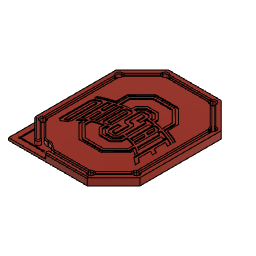
blockO_model (Autodesk Fusion 360 design; units mm, degrees)
Autodesk Fusion 360 part; units mm, degrees
(part 1 of 2)
sketch "Sketch1" plane through (0, 0, 0) normal (0, 0, 1) x (1, 0, 0)
  line L0 (0, 0) -> (25, 0)
  line L1 (0, 0) -> (-24, 24)
  line L2 (-24, 24) -> (-24, 104)
  line L3 (-24, 104) -> (0, 128)
  line L4 (0, 128) -> (25, 128)
  line L5 (25, 128) -> (25, 0) construction
  line L6 (50, 128) -> (25, 128)
  line L7 (74, 104) -> (50, 128)
  line L8 (74, 24) -> (74, 104)
  line L9 (50, 0) -> (74, 24)
  line L10 (50, 0) -> (25, 0)
  line L11 (0.4142, 127) -> (25, 127)
  line L12 (49.5858, 127) -> (25, 127)
  line L13 (73, 103.5858) -> (49.5858, 127)
  line L14 (73, 24.4142) -> (73, 103.5858)
  line L15 (49.5858, 1) -> (73, 24.4142)
  line L16 (49.5858, 1) -> (25, 1)
  line L17 (0.4142, 1) -> (25, 1)
  line L18 (0.4142, 1) -> (-23, 24.4142)
  line L19 (-23, 24.4142) -> (-23, 103.5858)
  line L20 (-23, 103.5858) -> (0.4142, 127)
  line L21 (50.4142, 129) -> (25, 129)
  line L22 (-0.4142, 129) -> (25, 129)
  line L23 (-25, 104.4142) -> (-0.4142, 129)
  line L24 (-25, 23.5858) -> (-25, 104.4142)
  line L25 (-0.4142, -1) -> (-25, 23.5858)
  line L26 (-0.4142, -1) -> (25, -1)
  line L27 (50.4142, -1) -> (25, -1)
  line L28 (50.4142, -1) -> (75, 23.5858)
  line L29 (75, 23.5858) -> (75, 104.4142)
  line L30 (75, 104.4142) -> (50.4142, 129)
  line L31 (-2.4853, 134) -> (25, 134)
  line L32 (52.4853, 134) -> (25, 134)
  line L33 (80, 106.4853) -> (52.4853, 134)
  line L34 (80, 21.5147) -> (80, 106.4853)
  line L35 (52.4853, -6) -> (80, 21.5147)
  line L36 (52.4853, -6) -> (25, -6)
  line L37 (-2.4853, -6) -> (25, -6)
  line L38 (-2.4853, -6) -> (-30, 21.5147)
  line L39 (-30, 21.5147) -> (-30, 106.4853)
  line L40 (-30, 106.4853) -> (-2.4853, 134)
  line L41 (-30, 21.5147) -> (-30, -6)
  line L42 (-30, -6) -> (-2.4853, -6)
  circle A0 centre (-24, 24) radius 2.5
  circle A1 centre (-24, 104) radius 2.5
  circle A2 centre (0, 128) radius 2.5
  circle A3 centre (50, 128) radius 2.5
  circle A4 centre (74, 104) radius 2.5
  circle A5 centre (74, 24) radius 2.5
  circle A6 centre (50, 0) radius 2.5
  circle A7 centre (0, 0) radius 6.4944
  line L43 (-4.5922, 4.5922) -> (-8.8348, 0.3496)
  line L44 (6.4944, 0) -> (6.4944, -6)
  line L45 (46.8934, 7.5) -> (25, 7.5)
  line L46 (3.1066, 7.5) -> (25, 7.5)
  line L47 (3.1066, 7.5) -> (-16.5, 27.1066)
  line L48 (-16.5, 27.1066) -> (-16.5, 100.8934)
  line L49 (-16.5, 100.8934) -> (3.1066, 120.5)
  line L50 (3.1066, 120.5) -> (25, 120.5)
  line L51 (46.8934, 120.5) -> (25, 120.5)
  line L52 (66.5, 100.8934) -> (46.8934, 120.5)
  line L53 (66.5, 27.1066) -> (66.5, 100.8934)
  line L54 (46.8934, 7.5) -> (66.5, 27.1066)
  line L55 (45.8579, 10) -> (25, 10)
  line L56 (4.1421, 10) -> (25, 10)
  line L57 (4.1421, 10) -> (-14, 28.1421)
  line L58 (-14, 28.1421) -> (-14, 99.8579)
  line L59 (-14, 99.8579) -> (4.1421, 118)
  line L60 (4.1421, 118) -> (25, 118)
  line L61 (45.8579, 118) -> (25, 118)
  line L62 (64, 99.8579) -> (45.8579, 118)
  line L63 (64, 28.1421) -> (64, 99.8579)
  line L64 (45.8579, 10) -> (64, 28.1421)
  line L65 (38.7955, 27.05) -> (25, 27.05)
  line L66 (11.2045, 27.05) -> (25, 27.05)
  line L67 (11.2045, 27.05) -> (3.05, 35.2045)
  line L68 (3.05, 35.2045) -> (3.05, 92.7955)
  line L69 (3.05, 92.7955) -> (11.2045, 100.95)
  line L70 (11.2045, 100.95) -> (25, 100.95)
  line L71 (38.7955, 100.95) -> (25, 100.95)
  line L72 (46.95, 92.7955) -> (38.7955, 100.95)
  line L73 (46.95, 35.2045) -> (46.95, 92.7955)
  line L74 (38.7955, 27.05) -> (46.95, 35.2045)
  line L75 (12.4885, 30.15) -> (25, 30.15)
  line L76 (37.5115, 30.15) -> (25, 30.15)
  line L77 (37.5115, 30.15) -> (43.85, 36.4885)
  line L78 (43.85, 36.4885) -> (43.85, 91.5115)
  line L79 (43.85, 91.5115) -> (37.5115, 97.85)
  line L80 (37.5115, 97.85) -> (25, 97.85)
  line L81 (12.4885, 97.85) -> (25, 97.85)
  line L82 (6.15, 91.5115) -> (12.4885, 97.85)
  line L83 (6.15, 36.4885) -> (6.15, 91.5115)
  line L84 (12.4885, 30.15) -> (6.15, 36.4885)
  line L85 (36.4759, 32.65) -> (25, 32.65)
  line L86 (13.5241, 32.65) -> (25, 32.65)
  line L87 (13.5241, 32.65) -> (8.65, 37.5241)
  line L88 (8.65, 37.5241) -> (8.65, 90.4759)
  line L89 (8.65, 90.4759) -> (13.5241, 95.35)
  line L90 (13.5241, 95.35) -> (25, 95.35)
  line L91 (36.4759, 95.35) -> (25, 95.35)
  line L92 (41.35, 90.4759) -> (36.4759, 95.35)
  line L93 (41.35, 37.5241) -> (41.35, 90.4759)
  line L94 (36.4759, 32.65) -> (41.35, 37.5241)
  line L95 (-23, 24.4142) -> (-25, 24.4142)
  line L96 (-25, 24.4142) -> (-23, 24.4142)
  line L97 (-23, 24.4142) -> (-23, 1)
  line L98 (-25, -1) -> (-25, 24.4142)
  line L99 (-0.4142, -1) -> (-25, -1)
  line L100 (-25, -1) -> (-25, 1)
  line L101 (-23, 1) -> (-0.4142, 1)
  line L102 (-0.4142, 1) -> (-0.4142, -1)
  line L103 (-24.5, -0.5) -> (-24.5, 23.9142)
  line L104 (-24.5, 23.9142) -> (-23.5, 23.9142)
  line L105 (-23.5, 23.9142) -> (-23.5, 0.5)
  line L106 (-23.5, 0.5) -> (-0.9142, 0.5)
  line L107 (-0.9142, 0.5) -> (-0.9142, -0.5)
  line L108 (-0.9142, -0.5) -> (-24.5, -0.5)
  line L109 (0, 0) -> (-51.0387, 0) construction
  line L110 (-24, 24) -> (-24, -3.1074) construction
  circle A8 centre (-24, 0) radius 1
  circle A9 centre (0, 0) radius 1.0824
  spline S0 degree 3 poles (-34.7934, -51.0937) (-33.9487, -51.2384) (-33.2949, -51.3375) (-32.4316, -51.4451) knots 0 0 0 0 1 1 1 1
  constraint coincident L0.start L1.start
  constraint horizontal L0
  constraint vertical L2
  constraint perpendicular L2 L4
  constraint symmetric L0.start L5 L9.start
  constraint symmetric L0.end L5 L10.end
  constraint symmetric L1.end L5 L8.start
  constraint symmetric L2.end L5 L7.start
  constraint symmetric L3.end L5 L6.start
  constraint symmetric L4.end L5 L6.end
  constraint perpendicular L37 L41
  constraint perpendicular L39 L42
  constraint coincident L1.end L2.start
  constraint coincident L2.end L3.start
  constraint coincident L3.end L4.start
  constraint coincident L6.start L7.end
  constraint coincident L7.start L8.end
  constraint coincident L8.start L9.end
  constraint coincident L9.start L10.start
  constraint equal A0 A1
  constraint equal A2 A3
  constraint equal A3 A4
  constraint equal A4 A5
  constraint equal A5 A6
  constraint coincident L37.start A7
  constraint coincident A7 L43.start
  constraint coincident L1 L43.start
  constraint coincident L38 L43.end
  constraint tangent A7 L43
  constraint coincident A7 L44.start
  constraint coincident L0 L44.start
  constraint coincident L37 L44.end
  constraint tangent A7 L44
  constraint equal A1 A2
  constraint coincident L24 L95.end
  constraint perpendicular L24 L95
  constraint horizontal L96
  constraint vertical L97
  constraint vertical L98
  constraint horizontal L99
  constraint vertical L100
  constraint horizontal L101
  constraint vertical L102
  constraint coincident L98 L100.end
  constraint collinear L17 L101
  constraint collinear L19 L97
  constraint perpendicular L98 L109
  constraint parallel L105 L110
  constraint coincident L109 A8.centre
  constraint coincident L110 A8.centre
  constraint tangent L99 A8
  constraint concentric A7 A9
  constraint coincident L101.end A9
extrude "Extrude1" add sketch "Sketch1" against normal blind 5 contours L17 L18 A7 | L26 A9 | L26 L37 L38 A7 L99 A9 | L25 L108 A9 | A7 L99 L108 A9 | L11 L12 L13 L14 L15 L16 L17 L18 L19 L20 A0 A1 A2 A3 A4 A5 A6 A7 | L26 L37 A7 L44 | L21 L22 L23 L24 L26 L27 L28 L29 L30 L31 L32 L33 L34 L35 L36 L37 L38 L39 L40 A0 A1 A2 A3 A4 A5 A6 L44 L98 | L25 L108 A9 | L38 A7 L99 L108 | L38 A7 L99 | L25 A7 L106 L108 A9 | L18 L19 A0 | L25 A7 L101 | L25 A7 L101 L106 | L38 A7 L43 L106 L108 | L15 L16 A6 | L27 L28 A6 | L25 A7 L43 L101 | L25 L38 L43 L97 L101 | A7 L43 L101 L106 | L25 L38 A0 L97 L105 | L38 L43 L101 L106 | L38 L43 L106 | L14 L15 A5 | L19 L20 A1 | L24 A0 L98 | L25 A0 L105 | L28 L29 A5 | L38 A0 L98 L103 | L25 A0 L98 L103 | L25 A0 L103 L105 | L38 A0 L103 L105 | L13 L14 A4 | L23 L24 A1 | L11 L20 A2 | L29 L30 A4 | L12 L13 A3 | L22 L23 A2 | L21 L30 A3 | L45 L46 L47 L48 L49 L50 L51 L52 L53 L54 | L55 L56 L57 L58 L59 L60 L61 L62 L63 L64 | L65 L66 L67 L68 L69 L70 L71 L72 L73 L74 | L75 L76 L77 L78 L79 L80 L81 L82 L83 L84 | L85 L86 L87 L88 L89 L90 L91 L92 L93 L94 makes body 1 at (9, 77.1953, -5) makes body 2 at (78.3333, 50.5286, -5)
sketch "Sketch3" plane through (0, 0, -5) normal (0, 0, -1) x (1, 0, 0)
  line L0 (49.5858, -1) -> (0.4142, -1)
  line L1 (0.4142, -1) -> (-23, -24.4142)
  line L2 (-23, -24.4142) -> (-23, -103.5858)
  line L3 (-23, -103.5858) -> (0.4142, -127)
  line L4 (0.4142, -127) -> (49.5858, -127)
  line L5 (49.5858, -127) -> (73, -103.5858)
  line L6 (73, -103.5858) -> (73, -24.4142)
  line L7 (73, -24.4142) -> (49.5858, -1)
  line L8 (52.4853, -134) -> (80, -106.4853)
  line L9 (-2.4853, -134) -> (52.4853, -134)
  line L10 (-30, -106.4853) -> (-2.4853, -134)
  line L11 (-30, -21.5147) -> (-30, -106.4853)
  line L12 (-2.4853, 6) -> (-30, -21.5147)
  line L13 (52.4853, 6) -> (-2.4853, 6)
  line L14 (80, -21.5147) -> (52.4853, 6)
  line L15 (80, -106.4853) -> (80, -21.5147)
  line L16 (-30, -21.5147) -> (-30, 6)
  line L17 (-30, 6) -> (-2.4853, 6)
  constraint coincident L11.start L12.end
  constraint perpendicular L13 L16
  constraint coincident L12.start L13.end
  constraint perpendicular L16 L17
extrude "Extrude2" add sketch "Sketch3" along normal blind 2.5 contours L0 L1 L2 L3 L4 L5 L6 L7 | L8 L9 L10 L11 L12 L13 L14 L15 bodies 1 2
extrude "Extrude3" add sketch "Sketch3" along normal blind 2.5 contours L12 L16 L17 bodies 1
sketch "Sketch4" plane through (0, 0, 0) normal (0, 0, 1) x (1, 0, 0)
extrude "Extrude4" cut sketch "Sketch1" against normal up to surface (5 mm away) contours L9 L10 L15 L16 A6 | L9 L10 L27 L28 A6 | L1 L18 A0 L97 | L18 L19 A0 | L15 L16 A6 | L27 L28 A6 | L2 L19 A0 L95 L96 | L1 L2 L95 L96 L97 L104 L105 | L1 A0 L97 | L2 L24 A0 L95 L96 | L1 L2 L24 L25 L95 L96 L98 L103 L104 | L1 L25 A0 L97 L105 | L8 L9 L14 L15 A5 | L8 L9 L28 L29 A5 | L14 L15 A5 | L2 L3 L19 L20 A1 | L19 L20 A1 | L24 A0 L98 | L1 L25 L103 L104 L105 | L1 L104 L105 | L25 A0 L105 | L28 L29 A5 | L2 L3 L23 L24 A1 | L25 A0 L98 L103 | L25 A0 L103 L105 | L13 L14 A4 | L7 L8 L13 L14 A4 | L23 L24 A1 | L7 L8 L29 L30 A4 | L3 L4 L11 L20 A2 | L11 L20 A2 | L29 L30 A4 | L12 L13 A3 | L6 L7 L12 L13 A3 | L3 L4 L22 L23 A2 | L22 L23 A2 | L6 L7 L21 L30 A3 | L21 L30 A3 bodies 1
extrude "Extrude5" cut sketch "Sketch1" against normal up to surface (5 mm away) contours L17 L18 A7 | L26 A9 | L26 L37 L38 A7 L99 A9 | L25 L108 A9 | A7 L99 L108 A9 | L26 L37 A7 L44 | L25 L108 A9 | L38 A7 L99 L108 | L38 A7 L99 | L25 A7 L106 L108 A9 | L25 A7 L101 | L25 A7 L101 L106 | L38 A7 L43 L106 L108 | L25 A7 L43 L101 | A7 L43 L101 L106 bodies 1
fillet "Fillet1" radius 7 2 edges at (-3.8303, 5.2445, -2.5) (6.4169, 1, -2.5) on bodies 1
fillet "Fillet2" radius 2.5 4 edges at (-5.2993, 3.8851, -2.5) (-8.8348, 0.3496, -2.5) (6.4944, -6, -2.5) (6.4944, -1, -2.5) on bodies 1
fillet "Fillet3" radius 2.5 28 edges at (-23, 26.2913, -2.5) (-21.6727, 23.0869, -2.5) (-25, 26.2913, -2.5) (-23.0869, 21.6727, -2.5) (-23.0869, 106.3273, -2.5) (-21.6727, 104.9131, -2.5) (-25, 101.7087, -2.5) (-23, 101.7087, -2.5) (2.2913, 129, -2.5) (-2.3273, 127.0869, -2.5) (-0.9131, 125.6727, -2.5) (2.2913, 127, -2.5) (52.3273, 127.0869, -2.5) (47.7087, 129, -2.5) (47.7087, 127, -2.5) (50.9131, 125.6727, -2.5) (73.0869, 106.3273, -2.5) (71.6727, 104.9131, -2.5) (73, 101.7087, -2.5) (75, 101.7087, -2.5) (73, 26.2913, -2.5) (71.6727, 23.0869, -2.5) (73.0869, 21.6727, -2.5) (75, 26.2913, -2.5) (50.9131, 2.3273, -2.5) (47.7087, 1, -2.5) (47.7087, -1, -2.5) (52.3273, 0.9131, -2.5) on bodies 1
fillet "Fillet4" radius 1 65 edges at (71.3147, 23.0049, 0) (71.6903, 24.9567, 0) (72.8049, 26.6025, 0) (73, 64, 0) (72.8049, 101.3975, 0) (71.6903, 103.0433, 0) (71.3147, 104.9951, 0) (61.2929, 115.2929, 0) (50.9951, 125.3147, 0) (49.0433, 125.6903, 0) (47.3975, 126.8049, 0) (25, 127, 0) (2.6025, 126.8049, 0) (0.9567, 125.6903, 0) (-0.9951, 125.3147, 0) (-11.2929, 115.2929, 0) (-21.3147, 104.9951, 0) (-21.6903, 103.0433, 0) (-22.8049, 101.3975, 0) (-23, 64, 0) (-22.8049, 26.6025, 0) (-21.6903, 24.9567, 0) (-21.3147, 23.0049, 0) (-13.8726, 15.2868, 0) (-4.2114, 6.6906, 0) (2.4853, 6, 0) (7.7089, 1.753, 0) (28.6483, 1, 0) (47.3975, 1.1951, 0) (49.0433, 2.3097, 0) (50.9951, 2.6853, 0) (61.2929, 12.7071, 0) (-20.3013, 11.816, 0) (-7.0671, 2.1173, 0) (-14.6247, 13.2104, 0) (-23.0049, 21.3147, 0) (-26.3097, 23.0433, 0) (-25.1951, 26.6025, 0) (-25, 64, 0) (-25.1951, 101.3975, 0) (-26.3097, 104.9567, 0) (-23.0049, 106.6853, 0) (-12.7071, 116.7071, 0) (-2.6853, 127.0049, 0) (-0.9567, 130.3097, 0) (2.6025, 129.1951, 0) (25, 129, 0) (47.3975, 129.1951, 0) (50.9567, 130.3097, 0) (52.6853, 127.0049, 0) (62.7071, 116.7071, 0) (73.0049, 106.6853, 0) (76.3097, 104.9567, 0) (75.1951, 101.3975, 0) (75, 64, 0) (75.1951, 26.6025, 0) (76.3097, 23.0433, 0) (73.0049, 21.3147, 0) (62.7071, 11.2929, 0) (52.6853, 0.9951, 0) (50.9567, -2.3097, 0) (47.3975, -1.1951, 0) (27.7118, -1, 0) (6.4944, -3.5, 0) (30.7398, -6, 0) on bodies 1
sketch "Sketch5" plane through (0, 0, 0) normal (0, 0, 1) x (-1, 0, 0)
  arc A0 (-70.0609, -22.8893) -> (-70.5002, -23.965) centre (-69.0003, -23.95) ccw
  arc A1 (-71.55, -26.4995) -> (-70.5002, -23.965) centre (-74, -24) ccw
  arc A2 (-71.55, -26.4995) -> (-72, -27.5707) centre (-70.5, -27.5707) ccw
  line L0 (-72, -27.5707) -> (-72, -100.4293)
  arc A3 (-72, -100.4293) -> (-71.55, -101.5005) centre (-70.5, -100.4293) ccw
  arc A4 (-70.5002, -104.035) -> (-71.55, -101.5005) centre (-74, -104) ccw
  arc A5 (-70.5002, -104.035) -> (-70.0609, -105.1107) centre (-69.0003, -104.05) ccw
  line L1 (-70.0609, -105.1107) -> (-51.1107, -124.0609)
  arc A6 (-51.1107, -124.0609) -> (-50.035, -124.5002) centre (-50.05, -123.0003) ccw
  arc A7 (-47.5005, -125.55) -> (-50.035, -124.5002) centre (-50, -128) ccw
  arc A8 (-47.5005, -125.55) -> (-46.4293, -126) centre (-46.4293, -124.5) ccw
  line L2 (-46.4293, -126) -> (-3.5707, -126)
  arc A9 (-3.5707, -126) -> (-2.4995, -125.55) centre (-3.5707, -124.5) ccw
  arc A10 (0.035, -124.5002) -> (-2.4995, -125.55) centre (0, -128) ccw
  arc A11 (0.035, -124.5002) -> (1.1107, -124.0609) centre (0.05, -123.0003) ccw
  line L3 (1.1107, -124.0609) -> (20.0609, -105.1107)
  arc A12 (20.0609, -105.1107) -> (20.5002, -104.035) centre (19.0003, -104.05) ccw
  arc A13 (21.55, -101.5005) -> (20.5002, -104.035) centre (24, -104) ccw
  arc A14 (21.55, -101.5005) -> (22, -100.4293) centre (20.5, -100.4293) ccw
  line L4 (22, -100.4293) -> (22, -27.5707)
  arc A15 (22, -27.5707) -> (21.55, -26.4995) centre (20.5, -27.5707) ccw
  arc A16 (20.5002, -23.965) -> (21.55, -26.4995) centre (24, -24) ccw
  arc A17 (20.5002, -23.965) -> (20.0609, -22.8893) centre (19.0003, -23.95) ccw
  line L5 (20.0609, -22.8893) -> (6.2701, -9.0985)
  arc A18 (6.2701, -9.0985) -> (1.126, -7.4093) centre (2.0275, -13.3412) ccw
  arc A19 (-6.0354, -4.443) -> (1.126, -7.4093) centre (0, 0) ccw
  arc A20 (-6.0354, -4.443) -> (-10.8673, -2) centre (-10.8673, -8) ccw
  line L6 (-10.8673, -2) -> (-46.4293, -2)
  arc A21 (-46.4293, -2) -> (-47.5005, -2.45) centre (-46.4293, -3.5) ccw
  arc A22 (-50.035, -3.4998) -> (-47.5005, -2.45) centre (-50, 0) ccw
  arc A23 (-50.035, -3.4998) -> (-51.1107, -3.9391) centre (-50.05, -4.9997) ccw
  line L7 (-51.1107, -3.9391) -> (-70.0609, -22.8893)
  line L8 (-108.9308, -166.2766) -> (-108.9012, -188.3914)
  line L9 (-108.9012, -188.3914) -> (-76.1248, -221.0889)
  line L10 (-76.1248, -221.0889) -> (-24.7372, -221.0889)
  line L11 (-24.7372, -221.0889) -> (8.4567, -188.4977)
  line L12 (8.4567, -188.4977) -> (8.4113, -166.3147)
  spline S0 degree 2 poles (8.4113, -166.3147) (24.5675, -160.7554) (37.454, -154.104) knots 0 0 0 1 1 1
  line L13 (37.454, -154.104) -> (37.5982, -69.2711)
  line L14 (37.5982, -69.2711) -> (27.8603, -62.9385)
  line L15 (27.8603, -62.9385) -> (14.9977, -70.6994)
  line L16 (14.9977, -70.6994) -> (9.072, -82.1954)
  line L17 (9.072, -82.1954) -> (-24.7992, -49.3035)
  line L18 (-24.7992, -49.3035) -> (-75.9426, -49.4418)
  line L19 (-75.9426, -49.4418) -> (-102.2338, -75.588)
  spline S1 degree 3 poles (-102.2338, -75.588) (-103.4051, -73.9683) (-105.3092, -72.9156) (-107.482, -72.9156) knots 0 0 0 0 1 1 1 1
  spline S2 degree 3 poles (-107.482, -72.9156) (-109.9076, -72.9156) (-112.0093, -74.237) (-113.1173, -76.1964) knots 0 0 0 0 1 1 1 1
  spline S3 degree 2 poles (-113.1173, -76.1964) (-120.0682, -70.9562) (-136.9942, -57.3225) knots 0 0 0 1 1 1
  line L20 (-136.9942, -57.3225) -> (-137.014, -154.3287)
  spline S4 degree 2 poles (-137.014, -154.3287) (-120.3333, -162.6226) (-108.9324, -166.2753) knots 0 0 0 1 1 1
  line L21 (-44.6848, -172.5597) -> (-40.0611, -168.0135)
  line L22 (-40.0611, -168.0135) -> (-40.0611, -137.1508)
  line L23 (-40.0611, -137.1508) -> (-45.0799, -132.3817)
  line L24 (-45.0799, -132.3817) -> (-53.5181, -132.3817)
  line L25 (-53.5181, -132.3817) -> (-53.5797, -104.2465)
  line L26 (-53.5797, -104.2465) -> (-46.7959, -104.2465)
  line L27 (-46.7959, -104.2465) -> (-46.7959, -123.1725)
  line L28 (-46.7959, -123.1725) -> (-40.0611, -123.1725)
  line L29 (-40.0611, -123.1725) -> (-40.0611, -102.4906)
  line L30 (-40.0611, -102.4906) -> (-44.6973, -97.9317)
  line L31 (-44.6973, -97.9317) -> (-55.9687, -97.8606)
  line L32 (-55.9687, -97.8606) -> (-60.545, -102.4905)
  line L33 (-60.545, -102.4905) -> (-60.4155, -135.4901)
  line L34 (-60.4155, -135.4901) -> (-55.4773, -140.2244)
  line L35 (-55.4773, -140.2244) -> (-46.9631, -140.218)
  line L36 (-46.9631, -140.218) -> (-46.941, -165.5468)
  line L37 (-46.941, -165.5468) -> (-53.7548, -165.5168)
  line L38 (-53.7548, -165.5168) -> (-53.7705, -149.2768)
  line L39 (-53.7705, -149.2768) -> (-60.4532, -149.2879)
  line L40 (-60.4532, -149.2879) -> (-60.4737, -168.035)
  line L41 (-60.4737, -168.035) -> (-55.9339, -172.5591)
  line L42 (-55.9339, -172.5591) -> (-44.6843, -172.5591)
  line L43 (-44.6843, -172.5591) -> (-44.6848, -172.5597)
  line L44 (-61.9499, -162.6549) -> (-61.9625, -156.2109)
  spline S5 degree 2 poles (-61.9625, -156.2109) (-63.7987, -156.0339) (-66.6067, -155.7179) knots 0 0 0 1 1 1
  line L45 (-66.6067, -155.7179) -> (-66.6004, -112.1784)
  spline S6 degree 3 poles (-66.6004, -112.1784) (-68.8917, -111.8466) (-71.2841, -111.5542) (-73.3668, -111.1845) knots 0 0 0 0 1 1 1 1
  line L46 (-73.3668, -111.1845) -> (-73.1556, -154.9169)
  spline S7 degree 2 poles (-73.1556, -154.9169) (-75.7123, -154.5566) (-78.0431, -154.1568) knots 0 0 0 1 1 1
  line L47 (-78.0431, -154.1568) -> (-78.0431, -160.6609)
  spline S8 degree 3 poles (-78.0431, -160.6609) (-72.4903, -161.6422) (-67.53, -162.1637) (-61.9453, -162.6567) knots 0 0 0 0 1 1 1 1
  line L48 (-61.9453, -162.6567) -> (-61.9499, -162.6549)
  spline S9 degree 3 poles (-30.7408, -161.8474) (-27.8253, -161.4571) (-24.8909, -161.1063) (-21.9484, -160.5564) knots 0 0 0 0 1 1 1 1
  line L49 (-21.9484, -160.5564) -> (-18.2902, -155.751)
  line L50 (-18.2902, -155.751) -> (-18.3455, -112.9846)
  line L51 (-18.3455, -112.9846) -> (-21.6576, -110.0059)
  spline S10 degree 3 poles (-21.6576, -110.0059) (-25.4027, -110.9082) (-28.2075, -111.3649) (-31.8243, -111.9196) knots 0 0 0 0 1 1 1 1
  line L52 (-31.8243, -111.9196) -> (-34.8567, -115.9064)
  line L53 (-34.8567, -115.9064) -> (-34.9926, -157.6681)
  line L54 (-34.9926, -157.6681) -> (-30.7404, -161.8477)
  line L55 (-30.7404, -161.8477) -> (-30.7408, -161.8474)
  line L56 (-83.6281, -159.6367) -> (-79.5512, -155.9059)
  line L57 (-79.5512, -155.9059) -> (-79.5576, -109.8445)
  spline S11 degree 3 poles (-79.5576, -109.8445) (-81.6165, -109.3104) (-83.6455, -108.89) (-85.6366, -108.2501) knots 0 0 0 0 1 1 1 1
  line L58 (-85.6366, -108.2501) -> (-85.6366, -131.2054)
  line L59 (-85.6366, -131.2054) -> (-89.6187, -130.0693)
  line L60 (-89.6187, -130.0693) -> (-89.6187, -106.8816)
  spline S12 degree 3 poles (-89.6187, -106.8816) (-91.6746, -106.1231) (-93.6877, -105.4641) (-95.6551, -104.595) knots 0 0 0 0 1 1 1 1
  line L61 (-95.6551, -104.595) -> (-95.6551, -151.4401)
  line L62 (-95.6551, -151.4401) -> (-92.1644, -157.7229)
  spline S13 degree 3 poles (-92.1644, -157.7229) (-89.1984, -158.5226) (-86.5958, -158.9982) (-83.6284, -159.6334) knots 0 0 0 0 1 1 1 1
  line L63 (-83.6284, -159.6334) -> (-83.6284, -159.6366)
  line L64 (-83.6284, -159.6366) -> (-83.6281, -159.6367)
  spline S14 degree 3 poles (-14.9753, -159.2291) (-12.9274, -158.7598) (-10.8779, -158.3647) (-8.8347, -157.8164) knots 0 0 0 0 1 1 1 1
  line L65 (-8.8347, -157.8164) -> (-8.7083, -106.2133)
  spline S15 degree 3 poles (-8.7083, -106.2133) (-10.772, -106.9054) (-12.6635, -107.5612) (-14.9579, -108.2469) knots 0 0 0 0 1 1 1 1
  line L66 (-14.9579, -108.2469) -> (-14.9753, -159.2291)
  spline S16 degree 3 poles (-5.4705, -156.9125) (-3.3451, -156.2978) (-1.2276, -155.8332) (0.8882, -155.051) knots 0 0 0 0 1 1 1 1
  line L67 (0.8882, -155.051) -> (0.8882, -134.0706)
  line L68 (0.8882, -134.0706) -> (5.0267, -132.484)
  line L69 (5.0267, -132.484) -> (5.101, -153.7785)
  spline S17 degree 3 poles (5.101, -153.7785) (7.2391, -153.0089) (9.2301, -152.4337) (11.3412, -151.5757) knots 0 0 0 0 1 1 1 1
  line L70 (11.3412, -151.5757) -> (11.3507, -96.2213)
  spline S18 degree 3 poles (11.3507, -96.2213) (9.1069, -97.7699) (7.3765, -98.6042) (4.6776, -100.2398) knots 0 0 0 0 1 1 1 1
  line L71 (4.6776, -100.2398) -> (4.7424, -125.5326)
  spline S19 degree 2 poles (4.7424, -125.5326) (2.3531, -126.5708) (0.5264, -127.1934) knots 0 0 0 1 1 1
  line L72 (0.5264, -127.1934) -> (0.4648, -102.4194)
  spline S20 degree 3 poles (0.4648, -102.4194) (-1.5926, -103.4197) (-3.3087, -104.0818) (-5.4641, -104.9935) knots 0 0 0 0 1 1 1 1
  line L73 (-5.4641, -104.9935) -> (-5.4704, -156.9128)
  line L74 (-5.4704, -156.9128) -> (-5.4705, -156.9125)
  line L75 (-97.7172, -156.2457) -> (-97.7172, -156.2425)
  line L76 (-97.7172, -156.2425) -> (-97.7409, -149.5267)
  spline S21 degree 2 poles (-97.7409, -149.5267) (-98.2118, -149.3924) (-102.7264, -147.9891) knots 0 0 0 1 1 1
  line L77 (-102.7264, -147.9891) -> (-102.7375, -101.568)
  spline S22 degree 3 poles (-102.7375, -101.568) (-104.9624, -100.4555) (-106.8871, -99.4125) (-108.8797, -98.1216) knots 0 0 0 0 1 1 1 1
  line L78 (-108.8797, -98.1216) -> (-108.8986, -145.8326)
  spline S23 degree 2 poles (-108.8986, -145.8326) (-114.3977, -143.7057) (-114.7959, -143.5302) knots 0 0 0 1 1 1
  line L79 (-114.7959, -143.5302) -> (-114.7959, -150.4594)
  spline S24 degree 3 poles (-114.7959, -150.4594) (-109.3158, -152.7917) (-103.3534, -154.522) (-97.7173, -156.246) knots 0 0 0 0 1 1 1 1
  line L80 (-97.7173, -156.246) -> (-97.7172, -156.2457)
  line L81 (-28.5871, -154.7729) -> (-28.7498, -117.9164)
  line L82 (-28.7498, -117.9164) -> (-24.4533, -117.1137)
  line L83 (-24.4533, -117.1137) -> (-24.5955, -154.1961)
  line L84 (-24.5955, -154.1961) -> (-28.5871, -154.7729)
  line L85 (-85.6953, -152.6001) -> (-85.6981, -152.6001)
  line L86 (-85.6981, -152.6001) -> (-89.4827, -151.6615)
  line L87 (-89.4827, -151.6615) -> (-89.4731, -136.8916)
  line L88 (-89.4731, -136.8916) -> (-85.6981, -137.8413)
  line L89 (-85.6981, -137.8413) -> (-85.6953, -152.6006)
  line L90 (-85.6953, -152.6006) -> (-85.6953, -152.6001)
  spline S25 degree 3 poles (-116.8488, -149.6405) (-116.8537, -149.6391) (-116.8598, -149.6376) (-116.8646, -149.6341) knots 0 0 0 0 1 1 1 1
  line L91 (-116.8646, -149.6341) -> (-116.8646, -149.6369)
  line L92 (-116.8646, -149.6369) -> (-116.8488, -149.6398)
  line L93 (-116.8488, -149.6398) -> (-116.8488, -149.6405)
  line L94 (-116.8646, -149.6341) -> (-117.0336, -79.2965)
  spline S26 degree 3 poles (-117.0336, -79.2965) (-121.6178, -75.8106) (-128.3494, -70.4788) (-132.5527, -66.9092) knots 0 0 0 0 1 1 1 1
  line L95 (-132.5527, -66.9092) -> (-132.5527, -75.3425)
  spline S27 degree 2 poles (-132.5527, -75.3425) (-129.6767, -77.6701) (-123.7666, -82.4359) knots 0 0 0 1 1 1
  line L96 (-123.7666, -82.4359) -> (-123.7666, -108.1013)
  spline S28 degree 2 poles (-123.7666, -108.1013) (-129.8504, -104.8003) (-132.5527, -103.1505) knots 0 0 0 1 1 1
  line L97 (-132.5527, -103.1505) -> (-132.5527, -111.1571)
  spline S29 degree 2 poles (-132.5527, -111.1571) (-129.9138, -112.8116) (-123.4984, -116.2153) knots 0 0 0 1 1 1
  line L98 (-123.4984, -116.2153) -> (-123.5141, -139.5594)
  spline S30 degree 2 poles (-123.5141, -139.5594) (-129.4715, -136.5981) (-132.5684, -134.8504) knots 0 0 0 1 1 1
  line L99 (-132.5684, -134.8504) -> (-132.5684, -142.2564)
  spline S31 degree 3 poles (-132.5684, -142.2564) (-127.5908, -145.1877) (-122.1074, -147.2799) (-116.8642, -149.6329) knots 0 0 0 0 1 1 1 1
  line L100 (-116.8642, -149.6329) -> (-116.8646, -149.6341)
  spline S32 degree 3 poles (20.027, -148.212) (23.3233, -146.6681) (26.4803, -145.2286) (29.641, -143.4588) knots 0 0 0 0 1 1 1 1
  line L101 (29.641, -143.4588) -> (32.8632, -137.3102)
  line L102 (32.8632, -137.3102) -> (32.8632, -71.6434)
  line L103 (32.8632, -71.6434) -> (27.7645, -68.227)
  spline S33 degree 3 poles (27.7645, -68.227) (26.9133, -68.7579) (18.9116, -73.6091) (18.4012, -73.8904) knots 0 0 0 0 1 1 1 1
  line L104 (18.4012, -73.8904) -> (15.4067, -80.306)
  line L105 (15.4067, -80.306) -> (15.3451, -144.7921)
  line L106 (15.3451, -144.7921) -> (20.0272, -148.2117)
  line L107 (20.0272, -148.2117) -> (20.027, -148.212)
  line L108 (21.6293, -140.3792) -> (21.634, -79.4451)
  line L109 (21.634, -79.4451) -> (26.3168, -76.2626)
  line L110 (26.3168, -76.2626) -> (26.2858, -137.9219)
  line L111 (26.2858, -137.9219) -> (21.6293, -140.3791)
  line L112 (21.6293, -140.3791) -> (21.6293, -140.3792)
  line L113 (-26.5537, -216.6516) -> (4.0133, -186.6401)
  line L114 (4.0133, -186.6401) -> (3.964, -163.089)
  spline S34 degree 3 poles (3.964, -163.089) (13.5084, -160.0334) (23.5174, -156.387) (32.766, -151.4072) knots 0 0 0 0 1 1 1 1
  line L115 (32.766, -151.4072) -> (32.766, -146.4444)
  spline S35 degree 3 poles (32.766, -146.4444) (22.5978, -152.3135) (7.4076, -157.3828) (-0.8384, -159.8041) knots 0 0 0 0 1 1 1 1
  line L116 (-0.8384, -159.8041) -> (-0.8384, -184.4267)
  line L117 (-0.8384, -184.4267) -> (-28.6497, -211.7754)
  line L118 (-28.6497, -211.7754) -> (-72.2251, -211.7847)
  line L119 (-72.2251, -211.7847) -> (-99.7125, -184.6162)
  line L120 (-99.7125, -184.6162) -> (-99.6786, -159.8943)
  spline S36 degree 3 poles (-99.6786, -159.8943) (-109.1898, -157.2219) (-123.4147, -151.8229) (-132.5753, -146.7128) knots 0 0 0 0 1 1 1 1
  line L121 (-132.5753, -146.7128) -> (-132.5753, -151.6787)
  spline S37 degree 3 poles (-132.5753, -151.6787) (-123.3662, -156.6255) (-114.2415, -159.9409) (-104.5042, -163.0557) knots 0 0 0 0 1 1 1 1
  line L122 (-104.5042, -163.0557) -> (-104.4734, -186.5518)
  line L123 (-104.4734, -186.5518) -> (-74.295, -216.6563)
  line L124 (-74.295, -216.6563) -> (-26.5586, -216.6563)
  line L125 (-26.5586, -216.6563) -> (-26.5537, -216.6516)
  line L126 (-41.0159, -181.851) -> (-30.8154, -171.8638)
  line L127 (-30.8154, -171.8638) -> (-30.8154, -165.9412)
  spline S38 degree 3 poles (-30.8154, -165.9412) (-32.5497, -166.1644) (-33.8962, -166.227) (-35.6146, -166.3949) knots 0 0 0 0 1 1 1 1
  line L128 (-35.6146, -166.3949) -> (-35.6146, -169.904)
  line L129 (-35.6146, -169.904) -> (-42.9228, -177.0362)
  line L130 (-42.9228, -177.0362) -> (-57.7617, -177.0362)
  line L131 (-57.7617, -177.0362) -> (-64.8974, -169.9378)
  line L132 (-64.8974, -169.9378) -> (-64.8974, -166.475)
  spline S39 degree 3 poles (-64.8974, -166.475) (-66.6159, -166.3131) (-68.018, -166.0997) (-69.7522, -165.8825) knots 0 0 0 0 1 1 1 1
  line L133 (-69.7522, -165.8825) -> (-69.7522, -171.8575)
  line L134 (-69.7522, -171.8575) -> (-59.7897, -181.851)
  line L135 (-59.7897, -181.851) -> (-41.0151, -181.851)
  line L136 (-41.0151, -181.851) -> (-41.0159, -181.851)
  line L137 (-65.0366, -108.6281) -> (-65.0366, -100.6651)
  line L138 (-65.0366, -100.6651) -> (-57.9072, -93.5266)
  line L139 (-57.9072, -93.5266) -> (-42.8676, -93.5019)
  line L140 (-42.8676, -93.5019) -> (-35.6242, -100.5419)
  line L141 (-35.6242, -100.5419) -> (-35.6242, -108.5943)
  spline S40 degree 3 poles (-35.6242, -108.5943) (-33.8781, -108.3691) (-32.5223, -108.3297) (-30.8156, -108.0295) knots 0 0 0 0 1 1 1 1
  line L142 (-30.8156, -108.0295) -> (-30.8156, -98.5732)
  line L143 (-30.8156, -98.5732) -> (-40.8831, -88.7092)
  line L144 (-40.8831, -88.7092) -> (-59.7471, -88.5703)
  line L145 (-59.7471, -88.5703) -> (-69.7836, -98.687)
  line L146 (-69.7836, -98.687) -> (-69.8083, -107.918)
  spline S41 degree 3 poles (-69.8083, -107.918) (-68.1017, -108.2104) (-66.7809, -108.4106) (-65.0369, -108.6279) knots 0 0 0 0 1 1 1 1
  line L147 (-65.0369, -108.6279) -> (-65.0366, -108.6281)
  spline S42 degree 3 poles (-0.8504, -99.0176) (4.1944, -96.5664) (7.728, -94.397) (11.3469, -91.746) knots 0 0 0 0 1 1 1 1
  line L148 (11.3469, -91.746) -> (11.3469, -86.0301)
  spline S43 degree 3 poles (11.3469, -86.0301) (9.1681, -87.7644) (6.4682, -90.0385) (4.0168, -91.4744) knots 0 0 0 0 1 1 1 1
  line L149 (4.0168, -91.4744) -> (4.0168, -84.212)
  line L150 (4.0168, -84.212) -> (-26.6326, -53.7407)
  line L151 (-26.6326, -53.7407) -> (-74.1063, -53.6944)
  line L152 (-74.1063, -53.6944) -> (-104.4699, -84.0797)
  line L153 (-104.4699, -84.0797) -> (-104.4699, -91.2)
  spline S44 degree 3 poles (-104.4699, -91.2) (-107.9008, -89.1418) (-110.9402, -87.0673) (-113.7629, -84.6693) knots 0 0 0 0 1 1 1 1
  line L154 (-113.7629, -84.6693) -> (-113.7629, -90.2833)
  spline S45 degree 3 poles (-113.7629, -90.2833) (-109.6287, -93.4437) (-104.9951, -96.5208) (-99.7231, -99.0172) knots 0 0 0 0 1 1 1 1
  line L155 (-99.7231, -99.0172) -> (-99.6953, -86.2124)
  line L156 (-99.6953, -86.2124) -> (-72.255, -58.513)
  line L157 (-72.255, -58.513) -> (-28.5212, -58.5376)
  line L158 (-28.5212, -58.5376) -> (-0.8486, -86.0582)
  line L159 (-0.8486, -86.0582) -> (-0.8486, -99.0179)
  line L160 (-0.8486, -99.0179) -> (-0.8504, -99.0176)
  line L161 (-30.4303, -207.3251) -> (-5.2451, -182.5272)
  line L162 (-5.2451, -182.5272) -> (-5.2451, -161.0222)
  spline S46 degree 3 poles (-5.2451, -161.0222) (-12.4132, -163.0272) (-19.2955, -164.2529) (-26.3868, -165.3214) knots 0 0 0 0 1 1 1 1
  line L163 (-26.3868, -165.3214) -> (-26.3868, -173.8118)
  line L164 (-26.3868, -173.8118) -> (-39.1516, -186.2618)
  line L165 (-39.1516, -186.2618) -> (-61.6444, -186.2618)
  line L166 (-61.6444, -186.2618) -> (-74.1627, -173.728)
  line L167 (-74.1627, -173.728) -> (-74.1627, -165.3763)
  spline S47 degree 3 poles (-74.1627, -165.3763) (-81.2498, -164.3334) (-88.094, -163.0255) (-95.2649, -161.0463) knots 0 0 0 0 1 1 1 1
  line L168 (-95.2649, -161.0463) -> (-95.2649, -182.4119)
  line L169 (-95.2649, -182.4119) -> (-70.3551, -207.3252)
  line L170 (-70.3551, -207.3252) -> (-30.4296, -207.3252)
  line L171 (-30.4296, -207.3252) -> (-30.4303, -207.3251)
  line L172 (-74.1971, -107.2773) -> (-74.1786, -96.824)
  line L173 (-74.1786, -96.824) -> (-61.7624, -84.1206)
  line L174 (-61.7624, -84.1206) -> (-39.05, -84.2842)
  line L175 (-39.05, -84.2842) -> (-26.3747, -96.7933)
  line L176 (-26.3747, -96.7933) -> (-26.3747, -107.21)
  spline S48 degree 3 poles (-26.3747, -107.21) (-18.8947, -105.7305) (-11.566, -103.6057) (-5.2886, -100.9015) knots 0 0 0 0 1 1 1 1
  line L177 (-5.2886, -100.9015) -> (-5.2886, -87.9481)
  line L178 (-5.2886, -87.9481) -> (-30.335, -63.2826)
  line L179 (-30.335, -63.2826) -> (-70.4513, -62.9709)
  line L180 (-70.4513, -62.9709) -> (-95.2809, -88.0659)
  line L181 (-95.2809, -88.0659) -> (-95.2837, -100.9207)
  spline S49 degree 3 poles (-95.2837, -100.9207) (-88.6804, -103.7177) (-81.9607, -105.7517) (-74.1976, -107.2785) knots 0 0 0 0 1 1 1 1
  line L182 (-74.1976, -107.2785) -> (-74.1971, -107.2773)
extrude "Extrude7" [suppressed]
extrude "Extrude8" [suppressed]
extrude "Extrude9" cut sketch "Sketch1" against normal blind 6 contours L0 L1 L102 A9 | L0 L1 L26 L102 A9 | L1 L25 L102 L106 L107 A9 | L1 L102 A9 | L26 A9 | L25 L108 A9 | L25 L106 A9 | L25 L106 L107 A9 | L25 L108 A9 | L25 A7 L106 L108 A9 | L38 A7 L43 L106 L108 | L38 L106 L108 A8 | L38 L43 L106 | L38 L103 L105 A8 bodies 1
extrude "Extrude10" cut sketch "Sketch1" against normal up to surface (7.5 mm away) contours L103 L108 A8 | L103 L105 L106 L108 A8 | L105 L106 A8 bodies 1
sketch "Sketch7" plane through (0, 0, 0) normal (0, 0, 1) x (-1, 0, 0)
  arc A0 (-70.0609, -22.8893) -> (-70.5002, -23.965) centre (-69.0003, -23.95) ccw
  arc A1 (-71.55, -26.4995) -> (-70.5002, -23.965) centre (-74, -24) ccw
  arc A2 (-71.55, -26.4995) -> (-72, -27.5707) centre (-70.5, -27.5707) ccw
  line L0 (-72, -27.5707) -> (-72, -100.4293)
  arc A3 (-72, -100.4293) -> (-71.55, -101.5005) centre (-70.5, -100.4293) ccw
  arc A4 (-70.5002, -104.035) -> (-71.55, -101.5005) centre (-74, -104) ccw
  arc A5 (-70.5002, -104.035) -> (-70.0609, -105.1107) centre (-69.0003, -104.05) ccw
  line L1 (-70.0609, -105.1107) -> (-51.1107, -124.0609)
  arc A6 (-51.1107, -124.0609) -> (-50.035, -124.5002) centre (-50.05, -123.0003) ccw
  arc A7 (-47.5005, -125.55) -> (-50.035, -124.5002) centre (-50, -128) ccw
  arc A8 (-47.5005, -125.55) -> (-46.4293, -126) centre (-46.4293, -124.5) ccw
  line L2 (-46.4293, -126) -> (-3.5707, -126)
  arc A9 (-3.5707, -126) -> (-2.4995, -125.55) centre (-3.5707, -124.5) ccw
  arc A10 (0.035, -124.5002) -> (-2.4995, -125.55) centre (0, -128) ccw
  arc A11 (0.035, -124.5002) -> (1.1107, -124.0609) centre (0.05, -123.0003) ccw
  line L3 (1.1107, -124.0609) -> (20.0609, -105.1107)
  arc A12 (20.0609, -105.1107) -> (20.5002, -104.035) centre (19.0003, -104.05) ccw
  arc A13 (21.55, -101.5005) -> (20.5002, -104.035) centre (24, -104) ccw
  arc A14 (21.55, -101.5005) -> (22, -100.4293) centre (20.5, -100.4293) ccw
  line L4 (22, -100.4293) -> (22, -27.5707)
  arc A15 (22, -27.5707) -> (21.55, -26.4995) centre (20.5, -27.5707) ccw
  arc A16 (20.5002, -23.965) -> (21.55, -26.4995) centre (24, -24) ccw
  arc A17 (20.5002, -23.965) -> (20.0609, -22.8893) centre (19.0003, -23.95) ccw
  line L5 (20.0609, -22.8893) -> (6.2701, -9.0985)
  arc A18 (6.2701, -9.0985) -> (1.126, -7.4093) centre (2.0275, -13.3412) ccw
  arc A19 (-6.0354, -4.443) -> (1.126, -7.4093) centre (0, 0) ccw
  arc A20 (-6.0354, -4.443) -> (-10.8673, -2) centre (-10.8673, -8) ccw
  line L6 (-10.8673, -2) -> (-46.4293, -2)
  arc A21 (-46.4293, -2) -> (-47.5005, -2.45) centre (-46.4293, -3.5) ccw
  arc A22 (-50.035, -3.4998) -> (-47.5005, -2.45) centre (-50, 0) ccw
  arc A23 (-50.035, -3.4998) -> (-51.1107, -3.9391) centre (-50.05, -4.9997) ccw
  line L7 (-51.1107, -3.9391) -> (-70.0609, -22.8893)
  line L8 (-54.159, -79.981) -> (-54.1443, -90.9277)
  line L9 (-54.1443, -90.9277) -> (-37.9201, -107.1128)
  line L10 (-37.9201, -107.1128) -> (-12.4834, -107.1128)
  line L11 (-12.4834, -107.1128) -> (3.9475, -90.9803)
  line L12 (3.9475, -90.9803) -> (3.925, -79.9998)
  spline S0 degree 2 poles (3.925, -79.9998) (11.9222, -77.248) (18.301, -73.9556) knots 0 0 0 1 1 1
  line L13 (18.301, -73.9556) -> (18.3724, -31.9636)
  line L14 (18.3724, -31.9636) -> (13.5521, -28.829)
  line L15 (13.5521, -28.829) -> (7.1852, -32.6706)
  line L16 (7.1852, -32.6706) -> (4.252, -38.3611)
  line L17 (4.252, -38.3611) -> (-12.5141, -22.0797)
  line L18 (-12.5141, -22.0797) -> (-37.8299, -22.1482)
  line L19 (-37.8299, -22.1482) -> (-50.8439, -35.0905)
  spline S1 degree 3 poles (-50.8439, -35.0905) (-51.4237, -34.2887) (-52.3662, -33.7676) (-53.4418, -33.7676) knots 0 0 0 0 1 1 1 1
  spline S2 degree 3 poles (-53.4418, -33.7676) (-54.6424, -33.7676) (-55.6828, -34.4217) (-56.2312, -35.3916) knots 0 0 0 0 1 1 1 1
  spline S3 degree 2 poles (-56.2312, -35.3916) (-59.6719, -32.7977) (-68.0502, -26.0491) knots 0 0 0 1 1 1
  line L20 (-68.0502, -26.0491) -> (-68.06, -74.0668)
  spline S4 degree 2 poles (-68.06, -74.0668) (-59.8031, -78.1723) (-54.1597, -79.9803) knots 0 0 0 1 1 1
  line L21 (-22.3574, -83.0911) -> (-20.0687, -80.8407)
  line L22 (-20.0687, -80.8407) -> (-20.0687, -65.5638)
  line L23 (-20.0687, -65.5638) -> (-22.553, -63.2031)
  line L24 (-22.553, -63.2031) -> (-26.7299, -63.2031)
  line L25 (-26.7299, -63.2031) -> (-26.7603, -49.2763)
  line L26 (-26.7603, -49.2763) -> (-23.4024, -49.2763)
  line L27 (-23.4024, -49.2763) -> (-23.4024, -58.6446)
  line L28 (-23.4024, -58.6446) -> (-20.0687, -58.6446)
  line L29 (-20.0687, -58.6446) -> (-20.0687, -48.4071)
  line L30 (-20.0687, -48.4071) -> (-22.3636, -46.1505)
  line L31 (-22.3636, -46.1505) -> (-27.9429, -46.1153)
  line L32 (-27.9429, -46.1153) -> (-30.2082, -48.4071)
  line L33 (-30.2082, -48.4071) -> (-30.144, -64.7418)
  line L34 (-30.144, -64.7418) -> (-27.6997, -67.0852)
  line L35 (-27.6997, -67.0852) -> (-23.4851, -67.0821)
  line L36 (-23.4851, -67.0821) -> (-23.4742, -79.6197)
  line L37 (-23.4742, -79.6197) -> (-26.847, -79.6049)
  line L38 (-26.847, -79.6049) -> (-26.8548, -71.5661)
  line L39 (-26.8548, -71.5661) -> (-30.1627, -71.5716)
  line L40 (-30.1627, -71.5716) -> (-30.1729, -80.8514)
  line L41 (-30.1729, -80.8514) -> (-27.9256, -83.0908)
  line L42 (-27.9256, -83.0908) -> (-22.3572, -83.0908)
  line L43 (-22.3572, -83.0908) -> (-22.3574, -83.0911)
  line L44 (-30.9036, -78.1883) -> (-30.9098, -74.9985)
  spline S5 degree 2 poles (-30.9098, -74.9985) (-31.8187, -74.9109) (-33.2087, -74.7544) knots 0 0 0 1 1 1
  line L45 (-33.2087, -74.7544) -> (-33.2055, -53.2026)
  spline S6 degree 3 poles (-33.2055, -53.2026) (-34.3397, -53.0383) (-35.524, -52.8936) (-36.5549, -52.7106) knots 0 0 0 0 1 1 1 1
  line L46 (-36.5549, -52.7106) -> (-36.4503, -74.3579)
  spline S7 degree 2 poles (-36.4503, -74.3579) (-37.7159, -74.1796) (-38.8696, -73.9817) knots 0 0 0 1 1 1
  line L47 (-38.8696, -73.9817) -> (-38.8696, -77.2012)
  spline S8 degree 3 poles (-38.8696, -77.2012) (-36.121, -77.687) (-33.6657, -77.9451) (-30.9013, -78.1891) knots 0 0 0 0 1 1 1 1
  line L48 (-30.9013, -78.1891) -> (-30.9036, -78.1883)
  spline S9 degree 3 poles (-15.4552, -77.7886) (-14.012, -77.5954) (-12.5595, -77.4217) (-11.103, -77.1495) knots 0 0 0 0 1 1 1 1
  line L49 (-11.103, -77.1495) -> (-9.2922, -74.7708)
  line L50 (-9.2922, -74.7708) -> (-9.3196, -53.6016)
  line L51 (-9.3196, -53.6016) -> (-10.959, -52.1272)
  spline S10 degree 3 poles (-10.959, -52.1272) (-12.8128, -52.5738) (-14.2012, -52.7999) (-15.9915, -53.0745) knots 0 0 0 0 1 1 1 1
  line L52 (-15.9915, -53.0745) -> (-17.4926, -55.0479)
  line L53 (-17.4926, -55.0479) -> (-17.5598, -75.7198)
  line L54 (-17.5598, -75.7198) -> (-15.455, -77.7887)
  line L55 (-15.455, -77.7887) -> (-15.4552, -77.7886)
  line L56 (-41.6342, -76.6943) -> (-39.6162, -74.8475)
  line L57 (-39.6162, -74.8475) -> (-39.6193, -52.0473)
  spline S11 degree 3 poles (-39.6193, -52.0473) (-40.6385, -51.7829) (-41.6428, -51.5748) (-42.6284, -51.2581) knots 0 0 0 0 1 1 1 1
  line L58 (-42.6284, -51.2581) -> (-42.6284, -62.6209)
  line L59 (-42.6284, -62.6209) -> (-44.5995, -62.0585)
  line L60 (-44.5995, -62.0585) -> (-44.5995, -50.5807)
  spline S12 degree 3 poles (-44.5995, -50.5807) (-45.6172, -50.2052) (-46.6137, -49.879) (-47.5875, -49.4488) knots 0 0 0 0 1 1 1 1
  line L61 (-47.5875, -49.4488) -> (-47.5875, -72.6369)
  line L62 (-47.5875, -72.6369) -> (-45.8597, -75.7469)
  spline S13 degree 3 poles (-45.8597, -75.7469) (-44.3915, -76.1427) (-43.1032, -76.3782) (-41.6343, -76.6926) knots 0 0 0 0 1 1 1 1
  line L63 (-41.6343, -76.6926) -> (-41.6343, -76.6942)
  line L64 (-41.6343, -76.6942) -> (-41.6342, -76.6943)
  spline S14 degree 3 poles (-7.6513, -76.4925) (-6.6376, -76.2602) (-5.6231, -76.0646) (-4.6117, -75.7932) knots 0 0 0 0 1 1 1 1
  line L65 (-4.6117, -75.7932) -> (-4.5492, -50.2498)
  spline S15 degree 3 poles (-4.5492, -50.2498) (-5.5707, -50.5924) (-6.507, -50.9171) (-7.6427, -51.2565) knots 0 0 0 0 1 1 1 1
  line L66 (-7.6427, -51.2565) -> (-7.6513, -76.4925)
  spline S16 degree 3 poles (-2.9465, -75.3458) (-1.8944, -75.0415) (-0.8463, -74.8115) (0.2011, -74.4244) knots 0 0 0 0 1 1 1 1
  line L67 (0.2011, -74.4244) -> (0.2011, -64.0391)
  line L68 (0.2011, -64.0391) -> (2.2496, -63.2538)
  line L69 (2.2496, -63.2538) -> (2.2864, -73.7945)
  spline S17 degree 3 poles (2.2864, -73.7945) (3.3447, -73.4135) (4.3303, -73.1288) (5.3753, -72.7041) knots 0 0 0 0 1 1 1 1
  line L70 (5.3753, -72.7041) -> (5.38, -45.3039)
  spline S18 degree 3 poles (5.38, -45.3039) (4.2693, -46.0704) (3.4128, -46.4834) (2.0768, -47.293) knots 0 0 0 0 1 1 1 1
  line L71 (2.0768, -47.293) -> (2.1088, -59.8129)
  spline S19 degree 2 poles (2.1088, -59.8129) (0.9262, -60.3268) (0.022, -60.6349) knots 0 0 0 1 1 1
  line L72 (0.022, -60.6349) -> (-0.0085, -48.3719)
  spline S20 degree 3 poles (-0.0085, -48.3719) (-1.027, -48.867) (-1.8764, -49.1948) (-2.9433, -49.6461) knots 0 0 0 0 1 1 1 1
  line L73 (-2.9433, -49.6461) -> (-2.9464, -75.3459)
  line L74 (-2.9464, -75.3459) -> (-2.9465, -75.3458)
  line L75 (-48.6082, -75.0157) -> (-48.6082, -75.0141)
  line L76 (-48.6082, -75.0141) -> (-48.62, -71.6898)
  spline S21 degree 2 poles (-48.62, -71.6898) (-48.8531, -71.6233) (-51.0878, -70.9287) knots 0 0 0 1 1 1
  line L77 (-51.0878, -70.9287) -> (-51.0933, -47.9504)
  spline S22 degree 3 poles (-51.0933, -47.9504) (-52.1946, -47.3998) (-53.1473, -46.8835) (-54.1336, -46.2445) knots 0 0 0 0 1 1 1 1
  line L78 (-54.1336, -46.2445) -> (-54.143, -69.8613)
  spline S23 degree 2 poles (-54.143, -69.8613) (-56.865, -68.8085) (-57.0621, -68.7216) knots 0 0 0 1 1 1
  line L79 (-57.0621, -68.7216) -> (-57.0621, -72.1515)
  spline S24 degree 3 poles (-57.0621, -72.1515) (-54.3495, -73.306) (-51.3981, -74.1625) (-48.6083, -75.0159) knots 0 0 0 0 1 1 1 1
  line L80 (-48.6083, -75.0159) -> (-48.6082, -75.0157)
  line L81 (-14.3891, -74.2867) -> (-14.4697, -56.0429)
  line L82 (-14.4697, -56.0429) -> (-12.3429, -55.6455)
  line L83 (-12.3429, -55.6455) -> (-12.4133, -74.0012)
  line L84 (-12.4133, -74.0012) -> (-14.3891, -74.2867)
  line L85 (-42.6574, -73.2112) -> (-42.6588, -73.2112)
  line L86 (-42.6588, -73.2112) -> (-44.5322, -72.7465)
  line L87 (-44.5322, -72.7465) -> (-44.5275, -65.4355)
  line L88 (-44.5275, -65.4355) -> (-42.6588, -65.9056)
  line L89 (-42.6588, -65.9056) -> (-42.6574, -73.2114)
  line L90 (-42.6574, -73.2114) -> (-42.6574, -73.2112)
  spline S25 degree 3 poles (-58.0783, -71.7461) (-58.0807, -71.7455) (-58.0838, -71.7448) (-58.0861, -71.743) knots 0 0 0 0 1 1 1 1
  line L91 (-58.0861, -71.743) -> (-58.0861, -71.7444)
  line L92 (-58.0861, -71.7444) -> (-58.0783, -71.7458)
  line L93 (-58.0783, -71.7458) -> (-58.0783, -71.7461)
  line L94 (-58.0861, -71.743) -> (-58.1698, -36.9262)
  spline S26 degree 3 poles (-58.1698, -36.9262) (-60.439, -35.2007) (-63.7711, -32.5614) (-65.8517, -30.7945) knots 0 0 0 0 1 1 1 1
  line L95 (-65.8517, -30.7945) -> (-65.8517, -34.9689)
  spline S27 degree 2 poles (-65.8517, -34.9689) (-64.4281, -36.1211) (-61.5026, -38.4802) knots 0 0 0 1 1 1
  line L96 (-61.5026, -38.4802) -> (-61.5026, -51.1844)
  spline S28 degree 2 poles (-61.5026, -51.1844) (-64.514, -49.5504) (-65.8517, -48.7338) knots 0 0 0 1 1 1
  line L97 (-65.8517, -48.7338) -> (-65.8517, -52.697)
  spline S29 degree 2 poles (-65.8517, -52.697) (-64.5454, -53.516) (-61.3698, -55.2008) knots 0 0 0 1 1 1
  line L98 (-61.3698, -55.2008) -> (-61.3776, -66.756)
  spline S30 degree 2 poles (-61.3776, -66.756) (-64.3265, -65.2902) (-65.8595, -64.4251) knots 0 0 0 1 1 1
  line L99 (-65.8595, -64.4251) -> (-65.8595, -68.0911)
  spline S31 degree 3 poles (-65.8595, -68.0911) (-63.3956, -69.542) (-60.6813, -70.5777) (-58.086, -71.7424) knots 0 0 0 0 1 1 1 1
  line L100 (-58.086, -71.7424) -> (-58.0861, -71.743)
  spline S32 degree 3 poles (9.6747, -71.0391) (11.3063, -70.2748) (12.8691, -69.5623) (14.4336, -68.6862) knots 0 0 0 0 1 1 1 1
  line L101 (14.4336, -68.6862) -> (16.0285, -65.6427)
  line L102 (16.0285, -65.6427) -> (16.0285, -33.1379)
  line L103 (16.0285, -33.1379) -> (13.5047, -31.4468)
  spline S33 degree 3 poles (13.5047, -31.4468) (13.0834, -31.7096) (9.1226, -34.1109) (8.8699, -34.2502) knots 0 0 0 0 1 1 1 1
  line L104 (8.8699, -34.2502) -> (7.3877, -37.4259)
  line L105 (7.3877, -37.4259) -> (7.3572, -69.3462)
  line L106 (7.3572, -69.3462) -> (9.6748, -71.0389)
  line L107 (9.6748, -71.0389) -> (9.6747, -71.0391)
  line L108 (10.4678, -67.1619) -> (10.4702, -36.9997)
  line L109 (10.4702, -36.9997) -> (12.7881, -35.4244)
  line L110 (12.7881, -35.4244) -> (12.7728, -65.9455)
  line L111 (12.7728, -65.9455) -> (10.4678, -67.1618)
  line L112 (10.4678, -67.1618) -> (10.4678, -67.1619)
  line L113 (-13.3826, -104.9164) -> (1.748, -90.0608)
  line L114 (1.748, -90.0608) -> (1.7236, -78.4031)
  spline S34 degree 3 poles (1.7236, -78.4031) (6.448, -76.8906) (11.4024, -75.0857) (15.9804, -72.6207) knots 0 0 0 0 1 1 1 1
  line L115 (15.9804, -72.6207) -> (15.9804, -70.1641)
  spline S35 degree 3 poles (15.9804, -70.1641) (10.9472, -73.0693) (3.4281, -75.5786) (-0.6536, -76.7771) knots 0 0 0 0 1 1 1 1
  line L116 (-0.6536, -76.7771) -> (-0.6536, -88.9652)
  line L117 (-0.6536, -88.9652) -> (-14.4201, -102.5027)
  line L118 (-14.4201, -102.5027) -> (-35.9897, -102.5073)
  line L119 (-35.9897, -102.5073) -> (-49.5959, -89.059)
  line L120 (-49.5959, -89.059) -> (-49.5791, -76.8218)
  spline S36 degree 3 poles (-49.5791, -76.8218) (-54.2871, -75.4989) (-61.3284, -72.8265) (-65.8629, -70.297) knots 0 0 0 0 1 1 1 1
  line L121 (-65.8629, -70.297) -> (-65.8629, -72.7551)
  spline S37 degree 3 poles (-65.8629, -72.7551) (-61.3044, -75.2037) (-56.7877, -76.8448) (-51.9678, -78.3866) knots 0 0 0 0 1 1 1 1
  line L122 (-51.9678, -78.3866) -> (-51.9525, -90.0171)
  line L123 (-51.9525, -90.0171) -> (-37.0144, -104.9187)
  line L124 (-37.0144, -104.9187) -> (-13.385, -104.9187)
  line L125 (-13.385, -104.9187) -> (-13.3826, -104.9164)
  line L126 (-20.5413, -87.6902) -> (-15.4921, -82.7466)
  line L127 (-15.4921, -82.7466) -> (-15.4921, -79.815)
  spline S38 degree 3 poles (-15.4921, -79.815) (-16.3506, -79.9254) (-17.0171, -79.9564) (-17.8677, -80.0395) knots 0 0 0 0 1 1 1 1
  line L128 (-17.8677, -80.0395) -> (-17.8677, -81.7765)
  line L129 (-17.8677, -81.7765) -> (-21.4852, -85.307)
  line L130 (-21.4852, -85.307) -> (-28.8304, -85.307)
  line L131 (-28.8304, -85.307) -> (-32.3626, -81.7933)
  line L132 (-32.3626, -81.7933) -> (-32.3626, -80.0792)
  spline S39 degree 3 poles (-32.3626, -80.0792) (-33.2132, -79.999) (-33.9072, -79.8934) (-34.7657, -79.7859) knots 0 0 0 0 1 1 1 1
  line L133 (-34.7657, -79.7859) -> (-34.7657, -82.7435)
  line L134 (-34.7657, -82.7435) -> (-29.8343, -87.6903)
  line L135 (-29.8343, -87.6903) -> (-20.5409, -87.6903)
  line L136 (-20.5409, -87.6903) -> (-20.5413, -87.6902)
  line L137 (-32.4314, -51.4452) -> (-32.4314, -47.5036)
  line L138 (-32.4314, -47.5036) -> (-28.9024, -43.97)
  line L139 (-28.9024, -43.97) -> (-21.4579, -43.9578)
  line L140 (-21.4579, -43.9578) -> (-17.8724, -47.4425)
  line L141 (-17.8724, -47.4425) -> (-17.8724, -51.4284)
  spline S40 degree 3 poles (-17.8724, -51.4284) (-17.0081, -51.317) (-16.337, -51.2975) (-15.4922, -51.1489) knots 0 0 0 0 1 1 1 1
  line L142 (-15.4922, -51.1489) -> (-15.4922, -46.468)
  line L143 (-15.4922, -46.468) -> (-20.4756, -41.5854)
  line L144 (-20.4756, -41.5854) -> (-29.8132, -41.5167)
  line L145 (-29.8132, -41.5167) -> (-34.7812, -46.5244)
  line L146 (-34.7812, -46.5244) -> (-34.7934, -51.0937)
  spline S41 degree 3 poles (-34.7934, -51.0937) (-33.9487, -51.2384) (-33.2949, -51.3375) (-32.4316, -51.4451) knots 0 0 0 0 1 1 1 1
  line L147 (-32.4316, -51.4451) -> (-32.4314, -51.4452)
  spline S42 degree 3 poles (-0.6595, -46.688) (1.8376, -45.4747) (3.5867, -44.4008) (5.3781, -43.0886) knots 0 0 0 0 1 1 1 1
  line L148 (5.3781, -43.0886) -> (5.3781, -40.2593)
  spline S43 degree 3 poles (5.3781, -40.2593) (4.2996, -41.1177) (2.9631, -42.2434) (1.7497, -42.9542) knots 0 0 0 0 1 1 1 1
  line L149 (1.7497, -42.9542) -> (1.7497, -39.3593)
  line L150 (1.7497, -39.3593) -> (-13.4216, -24.2761)
  line L151 (-13.4216, -24.2761) -> (-36.921, -24.2532)
  line L152 (-36.921, -24.2532) -> (-51.9508, -39.2938)
  line L153 (-51.9508, -39.2938) -> (-51.9508, -42.8183)
  spline S44 degree 3 poles (-51.9508, -42.8183) (-53.6491, -41.7995) (-55.1536, -40.7727) (-56.5508, -39.5857) knots 0 0 0 0 1 1 1 1
  line L154 (-56.5508, -39.5857) -> (-56.5508, -42.3646)
  spline S45 degree 3 poles (-56.5508, -42.3646) (-54.5044, -43.929) (-52.2108, -45.4521) (-49.6011, -46.6878) knots 0 0 0 0 1 1 1 1
  line L155 (-49.6011, -46.6878) -> (-49.5874, -40.3495)
  line L156 (-49.5874, -40.3495) -> (-36.0045, -26.6384)
  line L157 (-36.0045, -26.6384) -> (-14.3565, -26.6506)
  line L158 (-14.3565, -26.6506) -> (-0.6587, -40.2732)
  line L159 (-0.6587, -40.2732) -> (-0.6587, -46.6882)
  line L160 (-0.6587, -46.6882) -> (-0.6595, -46.688)
  line L161 (-15.3015, -100.2998) -> (-2.8349, -88.025)
  line L162 (-2.8349, -88.025) -> (-2.8349, -77.3801)
  spline S46 degree 3 poles (-2.8349, -77.3801) (-6.3831, -78.3725) (-9.7898, -78.9792) (-13.3, -79.5082) knots 0 0 0 0 1 1 1 1
  line L163 (-13.3, -79.5082) -> (-13.3, -83.7109)
  line L164 (-13.3, -83.7109) -> (-19.6185, -89.8736)
  line L165 (-19.6185, -89.8736) -> (-30.7523, -89.8736)
  line L166 (-30.7523, -89.8736) -> (-36.9488, -83.6694)
  line L167 (-36.9488, -83.6694) -> (-36.9488, -79.5354)
  spline S47 degree 3 poles (-36.9488, -79.5354) (-40.4569, -79.0191) (-43.8448, -78.3717) (-47.3944, -77.392) knots 0 0 0 0 1 1 1 1
  line L168 (-47.3944, -77.392) -> (-47.3944, -87.9679)
  line L169 (-47.3944, -87.9679) -> (-35.0641, -100.2999)
  line L170 (-35.0641, -100.2999) -> (-15.3011, -100.2999)
  line L171 (-15.3011, -100.2999) -> (-15.3015, -100.2998)
  line L172 (-36.9659, -50.7766) -> (-36.9567, -45.6022)